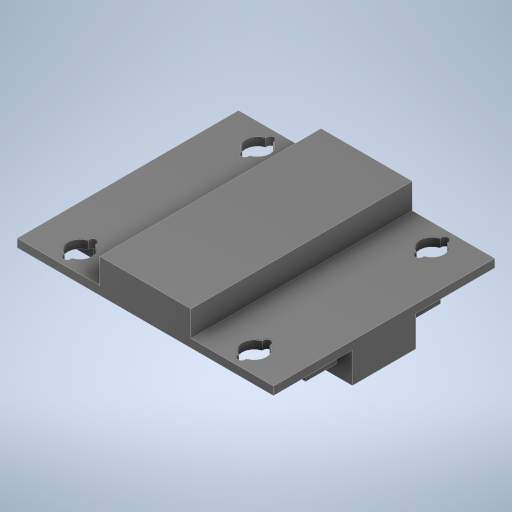
# Autodesk Inventor part: SUSTAINA-STRAINGAUGE-SENSING-BOARD
Saved by Autodesk Inventor 2024.2 (Build 282272000, 272)
## iProperties
Created: 2023-04-23
Part Number: SUSTAINA-STRAINGAUGE-SENSING-BOARD
Material: Acetal Resin, Black
Document SubType Name: Modeling
Designer: Masato Kubotera
Appearance: Smooth - Black
Description: Electrical Component
Surface Area: 66.2423 cm^2
Volume: 11.6813 cm^3
Vendor: JLCPCB
Author: Masato Kubotera
Autodesk Inventor part; units mm, degrees
ref_plane "YZ Plane" through (0, 0, 0) normal (1, 0, 0) x (0, 1, 0)
ref_plane "XZ Plane" through (0, 0, 0) normal (0, 1, 0) x (-1, 0, 0)
ref_plane "XY Plane" through (0, 0, 0) normal (0, 0, 1) x (1, 0, 0)
sketch "スケッチ1" plane through (0, 0, 0) normal (0, 0, 1) x (1, 0, 0)
  line L0 (-25, -21.59) -> (25, -21.59)
  line L1 (25, -21.59) -> (25, 21.59)
  line L2 (25, 21.59) -> (-25, 21.59)
  line L3 (-25, 21.59) -> (-25, -21.59)
  line L4 (-25, -21.59) -> (25, 21.59) construction
  line L5 (25, -21.59) -> (-25, 21.59) construction
  line L6 (-17, -17.34) -> (17, -17.34) construction
  line L7 (17, -17.34) -> (17, 17.34) construction
  line L8 (17, 17.34) -> (-17, 17.34) construction
  line L9 (-17, 17.34) -> (-17, -17.34) construction
  line L10 (-17, -17.34) -> (17, 17.34) construction
  line L11 (17, -17.34) -> (-17, 17.34) construction
  line L12 (-25, 6.2) -> (-10, 6.2)
  line L13 (-10, 6.2) -> (-10, -6.2)
  line L14 (-10, -6.2) -> (-25, -6.2)
  line L15 (-25, 0) -> (25, 0) construction
  line L16 (0, -21.59) -> (0, 21.59) construction
  line L17 (25, 6.2) -> (10, 6.2)
  line L18 (10, 6.2) -> (10, -6.2)
  line L19 (10, -6.2) -> (25, -6.2)
  line L20 (-8.89, -21.59) -> (8.89, -21.59)
  line L21 (8.89, -21.59) -> (8.89, 21.59)
  line L22 (8.89, 21.59) -> (-8.89, 21.59)
  line L23 (-8.89, 21.59) -> (-8.89, -21.59)
  line L24 (-8.89, -21.59) -> (8.89, 21.59) construction
  line L25 (8.89, -21.59) -> (-8.89, 21.59) construction
  circle A0 centre (17, 17.34) radius 2.4
  arc A1 (16.2801, 15.0505) -> (17.7199, 15.0505) centre (17, 14.84) ccw
  arc A2 (17.7199, 19.6295) -> (16.2801, 19.6295) centre (17, 19.84) ccw
  circle A3 centre (-17, 17.34) radius 2.4
  arc A4 (-16.2801, 19.6295) -> (-17.7199, 19.6295) centre (-17, 19.84) ccw
  arc A5 (-17.7199, 15.0505) -> (-16.2801, 15.0505) centre (-17, 14.84) ccw
  circle A6 centre (17, -17.34) radius 2.4
  arc A7 (16.2801, -19.6295) -> (17.7199, -19.6295) centre (17, -19.84) ccw
  arc A8 (17.7199, -15.0505) -> (16.2801, -15.0505) centre (17, -14.84) ccw
  circle A9 centre (-17, -17.34) radius 2.4
  arc A10 (-16.2801, -15.0505) -> (-17.7199, -15.0505) centre (-17, -14.84) ccw
  arc A11 (-17.7199, -19.6295) -> (-16.2801, -19.6295) centre (-17, -19.84) ccw
  line L26 (-22.86, -13.16) -> (-18.61, -13.16)
  line L27 (-18.61, -13.16) -> (-18.61, -7.16)
  line L28 (-18.61, -7.16) -> (-22.86, -7.16)
  line L29 (-22.86, -7.16) -> (-22.86, -13.16)
  line L30 (-22.86, -13.16) -> (-18.61, -7.16) construction
  line L31 (-18.61, -13.16) -> (-22.86, -7.16) construction
  line L32 (-22.86, 13.16) -> (-18.61, 13.16)
  line L33 (-18.61, 13.16) -> (-18.61, 7.16)
  line L34 (-18.61, 7.16) -> (-22.86, 7.16)
  line L35 (-22.86, 7.16) -> (-22.86, 13.16)
  line L36 (22.86, -13.16) -> (18.61, -13.16)
  line L37 (18.61, -13.16) -> (18.61, -7.16)
  line L38 (18.61, -7.16) -> (22.86, -7.16)
  line L39 (22.86, -7.16) -> (22.86, -13.16)
  line L40 (18.61, 13.16) -> (18.61, 7.16)
  line L41 (22.86, 13.16) -> (18.61, 13.16)
  line L42 (22.86, 7.16) -> (22.86, 13.16)
  line L43 (18.61, 7.16) -> (22.86, 7.16)
  point P0 (0, 0)
  point P1 (-10, 0)
  point P2 (25, 6.2)
  point P3 (25, -6.2)
  point P4 (0, 0)
  point P5 (0, 0)
  point P6 (0, 0)
  point P7 (17, 20.59)
  point P8 (17, 14.09)
  point P9 (-20.735, -10.16)
  point P10 (-22.86, -10.16)
  dimension "d0" = 50
  dimension "d1" = 43.18
  dimension "d2" = 34
  dimension "d3" = 34.68
  dimension "d8" = 15
  dimension "d9" = 12.4
  dimension "d17" = 17.78
  dimension "d18" = 43.18
  dimension "d25" = 16
  dimension "d26" = 4.8
  dimension "d27" = 6.5
  dimension "d28" = 1.5
  dimension "d29" = 1
  dimension "d30" = 8.5
  dimension "d31" = 16
  dimension "d32" = 4.25
  dimension "d33" = 6
  dimension "d34" = 10.16
  dimension "d35" = 22.86
  constraints: 88 end point, 37 symmetric about line, 34 point on circle, 18 midpoint, 12 centre point, 8 parallel, 7 perpendicular, 4 coincident, 4 horizontal, 3 point on line, 11 other
  measures "d0" distance of L2.end L1.end
  measures "d1" distance of L1.end L0.end
  measures "d2" distance of L8.end L7.end
  measures "d3" distance of L6.end L7.end
  measures "d8" distance of L12.start L12.end
  measures "d9" distance of L12.end L13.end
  measures "d17" distance of L22.end L21.end
  measures "d18" distance of L21.end L20.end
  measures "d25" diameter of L3 L9
  measures "d26" diameter of A0
  measures "d27" distance of point (17, 20.59) point (17, 14.09)
  measures "d28" diameter of A1
  measures "d29" distance from line of point (17, 20.59) L2
  measures "d30" diameter of L2 L8
  measures "d31" diameter of L1 L7
  measures "d32" distance of L28.end L27.end
  measures "d33" distance of L27.end L26.end
  measures "d34" distance from line of point (-22.86, -10.16) L15
  measures "d35" distance from line of point (-22.86, -10.16) L16
extrude "押し出し1" add sketch "スケッチ1" along normal blind 1.6 contours L3 L14 L13 L12 L2 L23 L0 | L23 L2 L21 L0 | L3 L12 L13 L14 | L21 L2 L1 L17 L18 L19 L0 | L19 L18 L17 L1 | L29 L28 L27 L26 | L32 L33 L34 L35 | L36 L37 L38 L39 | L41 L42 L43 L40
extrude "押し出し2" add sketch "スケッチ1" against normal blind 6 contours L3 L12 L13 L14 | L19 L18 L17 L1
extrude "押し出し3" add sketch "スケッチ1" along normal blind 6.6 contours L23 L2 L21 L0
extrude "Extrusion4" add sketch "スケッチ1" against normal blind 2.9 contours L29 L28 L27 L26 | L32 L33 L34 L35 | L36 L37 L38 L39 | L41 L42 L43 L40
